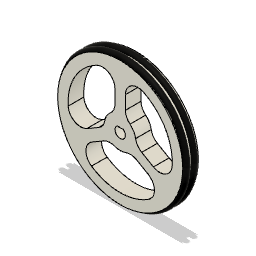
Roda Nema 17 v7 (Autodesk Fusion 360 design; units mm, degrees)
Autodesk Fusion 360 part; units mm, degrees
sketch "Sketch1" plane through (0, 0, 0) normal (0, 0, 1) x (1, 0, 0)
  circle A0 centre (0, 0) radius 7.5
  line L0 (-1.51, 2) -> (1.51, 2)
  arc A1 (-1.51, 2) -> (1.51, 2) centre (0, 0) ccw
  dimension "d3" = 15
  dimension "d4" = 5.012
  dimension "d5" = 2
  constraint coincident A0.centre A1.centre
  constraint horizontal L0
  measures "d3" diameter of A0
  measures "d4" diameter of A1
  measures "d5" distance of A0.centre L0
sketch "Sketch2" plane through (0, 0, 0) normal (0, 0, 1) x (1, 0, 0)
  circle A0 centre (0, 0) radius 25
  circle A1 centre (0, 0) radius 30
  point P0 (0, 30)
  dimension "d8" = 5
  dimension "d9" = 60
  constraint coincident A0.centre A1.centre
  constraint concentric A0 A1
  constraint vertical A0.centre P0
  constraint coincident A1 P0
  measures "d8" distance of A0 A1
  measures "d9" diameter of A1
sketch "Sketch3" plane through (0, 0, 0) normal (0, 0, 1) x (1, 0, 0)
  line L0 (-2.5, 7.0711) -> (-2.5, 24.8747)
  line L1 (2.5, 7.0711) -> (2.5, 24.8747)
  circle A0 centre (0, 0) radius 7.5
  circle A1 centre (0, 0) radius 25
  line L2 (-2.5, 15.9729) -> (2.5, 15.9729) construction
  arc A2 (2.5, 24.8747) -> (-2.5, 24.8747) centre (0, 0) ccw
  arc A3 (2.5, 7.0711) -> (-2.5, 7.0711) centre (0, 0) ccw
  point P0 (0, 15.9729)
  dimension "d10" = 5
  constraint vertical L0
  constraint vertical L1
  constraint coincident L0.start A0
  constraint coincident L1.start A0
  constraint coincident L1.end A1
  constraint coincident L0.end A1
  constraint midpoint L0 L2.start
  constraint coincident L1 L2.end
  constraint perpendicular L1 L2
  constraint midpoint L2 P0
  constraint vertical P0 A0.centre
  constraint coincident A0.centre A1.centre
  measures "d10" distance of L0 L1
extrude "Extrude2" add sketch "Sketch1" sketch "Sketch2" along normal mid plane 7.5 of sketch 2 makes body 1 at (7.4627, -0.7468, 2.5) makes body 2 at (28.2216, -1.4904, 3.75)
extrude "Extrude3" add sketch "Sketch3" along normal mid plane 7.5 contours L0 L1 A0 A1 A2 A3 bodies 1 2
pattern_circular "C-Pattern1" count 3 over 360 about axis through (0, 0, 0) along (0, 0, 1) of "Extrude3"
sketch "Sketch4" plane through (0, 0, 0) normal (1, 0, 0) x (0, 0, -1)
  line L0 (-3.75, 30) -> (-2.25, 28.75)
  line L1 (-2.25, 28.75) -> (2.25, 28.75)
  line L2 (2.25, 28.75) -> (3.75, 30)
  line L3 (3.75, 30) -> (-3.75, 30)
  line L4 (-3.75, 30) -> (-3.75, -30)
  line L5 (0, 30) -> (0, -30)
  point P0 (0, 30)
  point P1 (0, 28.75)
  dimension "d19" = 1.25
  dimension "d20" = 1.5
  constraint horizontal L1
  constraint parallel L1 L3
  constraint midpoint L3 P0
  constraint coincident L0.start L4
  constraint midpoint L1 P1
  constraint coincident P1 L5
  measures "d19" distance of L1 L3
  measures "d20" distance of L0.end L4
revolve "Revolve2" cut sketch "Sketch4" angle 360 about axis through (0, 0, 0) along (0, 0, -1) bodies 1
fillet "Fillet1" radius 6 12 edges at (7.3737, -1.3705, 0) (2.5, 7.0711, 0) (-2.5, 7.0711, 0) (-7.3737, -1.3705, 0) (-4.8737, -5.7006, 0) (4.8737, -5.7006, 0) (-2.5, 24.8747, 0) (2.5, 24.8747, 0) (-22.7921, -10.2723, 0) (22.7921, -10.2723, 0) (20.2921, -14.6024, 0) (-20.2921, -14.6024, 0) on bodies 1
fillet "Fillet1" radius 1 2 edges at (-26.8044, 10.3964, -2.25) (-26.8044, 10.3964, 2.25) on bodies 1
sketch "Sketch5" plane through (0, 0, 0) normal (1, 0, 0) x (0, 0, -1)
  circle A0 centre (-1.8031, 30) radius 1.25
  line L0 (3.75, 30) -> (-3.75, 30)
  point P0 (-1.888, 28.75)
  point P1 (-2.5281, 28.9818)
  dimension "d29" = 2.5
  constraint coincident A0.centre L0
  constraint coincident A0 P1
  measures "d29" diameter of A0
revolve "Revolve3" add sketch "Sketch5" angle 360 about axis through (0, 0, 2.25) along (0, 0, -1) separate body makes body 3
mirror "Mirror1" about plane through (0, 0, 0) normal (0, 0, 1) of bodies 3 makes body 4
equation "d9 = diametro"
equation "espessura = 7.5 mm"
equation "diametro = 60 mm"
equation "d13 = espessura"
equation "d15 = espessura"
